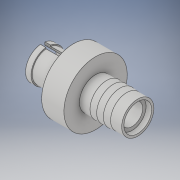
# Autodesk Inventor part: ARTHURW5.5a AXLE
Saved by Autodesk Inventor 2018 (Build 220112000, 112)
## iProperties
Created: 2019-01-18
Part Number: ARTHURW5.5a AXLE
Material: Generic
Document SubType Name: Modeling
Designer: This kid
Density: 1 g/cm^3
Appearance: Default
Author: This kid
Autodesk Inventor part; units mm, degrees
ref_plane "YZ Plane" through (0, 0, 0) normal (1, 0, 0) x (0, 1, 0)
ref_plane "XZ Plane" through (0, 0, 0) normal (0, 1, 0) x (-1, 0, 0)
ref_plane "XY Plane" through (0, 0, 0) normal (0, 0, 1) x (1, 0, 0)
sketch "Sketch1" plane through (0, 0, 0) normal (0, 0, 1) x (1, 0, 0)
  line L0 (0, 0) -> (0, 2.413)
  line L1 (0, 2.413) -> (-4.826, 2.413)
  line L2 (-4.826, 2.413) -> (-4.826, 3.175)
  line L3 (-4.826, 3.175) -> (-11.176, 3.175)
  line L4 (-11.176, 3.175) -> (-11.176, 3.81)
  line L5 (-11.176, 3.81) -> (-9.906, 3.81)
  line L6 (-9.906, 3.81) -> (-9.906, 3.556)
  line L7 (-9.906, 3.556) -> (0.254, 3.6741)
  line L8 (0.254, 3.6741) -> (0.254, 5.842)
  line L9 (0.254, 5.842) -> (-4.064, 5.842)
  line L10 (-4.064, 5.842) -> (-4.064, 7.239)
  line L11 (-4.064, 7.239) -> (1.016, 7.239)
  line L12 (1.016, 7.239) -> (1.016, 3.683)
  line L13 (1.016, 3.683) -> (3.556, 3.683)
  line L14 (3.556, 3.683) -> (3.556, 3.81)
  line L15 (3.556, 3.81) -> (5.08, 3.683)
  line L16 (5.08, 3.683) -> (5.08, 3.81)
  line L17 (5.08, 3.81) -> (6.604, 3.683)
  line L18 (6.604, 3.683) -> (6.604, 3.81)
  line L19 (6.604, 3.81) -> (8.128, 3.683)
  line L20 (8.128, 3.683) -> (10.668, 3.683)
  line L21 (10.668, 3.683) -> (10.668, 3.175)
  line L22 (10.668, 3.175) -> (9.398, 3.175)
  line L23 (9.398, 3.175) -> (9.398, 2.413)
  line L24 (9.398, 2.413) -> (1.057, 2.413)
  line L25 (1.057, 2.413) -> (1.057, 0)
  line L26 (1.057, 0) -> (0, 0)
  dimension "d0" = 21.844
  dimension "d1" = 1.27
  dimension "d2" = 6.35
  dimension "d3" = 11.43
  dimension "d4" = 5.08
  dimension "d5" = 1.524
  dimension "d6" = 1.524
  dimension "d7" = 1.524
  dimension "d8" = 1.27
  dimension "d9" = 2.54
  dimension "d10" = 2.54
  dimension "d11" = 4.826
  dimension "d13" = 5.842
  dimension "d14" = 7.239
  dimension "d15" = 0.254
  dimension "d16" = 0.127
  dimension "d17" = 0.127
  dimension "d18" = 2.413
  dimension "d19" = 3.175
  dimension "d20" = 3.683
  dimension "d21" = 3.81
  dimension "d22" = 3.175
  dimension "d23" = 2.413
  constraints: 54 end point, 16 perpendicular, 3 horizontal, 3 parallel, 3 point on line, 2 vertical
  measures "d0" distance between parallel lines of L21 L4
  measures "d1" distance of L4.end L5.end
  measures "d2" distance of L2.end L3.end
  measures "d3" distance from line of L8 L4.end
  measures "d4" distance of L10.end L11.end
  measures "d5" distance of L15.end L13.end
  measures "d6" distance of L15.end L17.end
  measures "d7" distance of L17.end L19.end
  measures "d8" distance from line of L21.end L23
  measures "d9" distance of L19.end L20.end
  measures "d10" distance of L12.end L13.end
  measures "d11" distance between parallel lines of L0 L2
  measures "d13" distance between parallel lines of L26 L9
  measures "d14" distance between parallel lines of L11 L26
  measures "d15" distance of L5.end L6.end
  measures "d16" distance of L13.end L14.end
  measures "d17" distance of L15.end L16.end
  measures "d18" vertical distance of L23.end L25.end
  measures "d19" distance from line of L26 L21.end
  measures "d20" distance from line of L20.end L26
  measures "d21" distance from line of L4.end L26
  measures "d22" distance from line of L0.start L3
  measures "d23" distance from line of L0.start L1
revolve "Revolution1" add sketch "Sketch1" angle 360 about axis through (1.057, 0, 0) along (-1, 0, 0)
sketch "Sketch2" plane through (-11.176, 0, 0) normal (-1, 0, 0) x (0, 0, 1)
  circle A0 centre (0, 0) radius 3.81 projected
  line L0 (0.4164, -4.7623) -> (-0.5996, -4.7623)
  line L1 (-0.5996, -4.7623) -> (-0.5996, 4.4311)
  line L2 (-0.5996, 4.4311) -> (0.4164, 4.4311)
  line L3 (0.4164, 4.4311) -> (0.4164, -4.7623)
  dimension "d25" = 1.016
  constraints: 8 end point, 2 parallel, 1 horizontal, 1 perpendicular
  measures "d25" distance of L1.end L2.end
extrude "Extrusion1" cut sketch "Sketch2" against normal blind 5.08 contours L3 A0 L1 | A0 L1 L2 L3 | L3 L0 L1 A0
equation "\"d6\" = d5"
equation "\"d7\" = d6"
body "Solid1"
